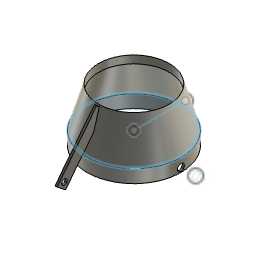
rudder (Autodesk Fusion 360 design; units mm, degrees)
Autodesk Fusion 360 part; units mm, degrees
note: some values were not read from the file. Chosen so that the rebuilt part matches the saved one: which bodies a step acts on.
sketch "Sketch1" plane through (0, 0, 0) normal (0, 0, 1) x (1, 0, 0) in component "Steering"
  circle A0 centre (-250, 0) radius 22
  line L0 (-250, 0) -> (-250, 24)
  circle A1 centre (-250, 0) radius 21
  dimension "d1" = 44
  dimension "d31" = 42
  constraint coincident A0.centre L0.start
  constraint vertical L0
  constraint concentric A0 A1
  measures "d1" diameter of A0
  measures "d31" diameter of A1
ref_plane "WorkPlane1" through (-225, 0, 0) normal (1, 0, 0) x (0, 1, 0) in component "Steering"
box "BoxPrimitive1" add length 30 width 1 height 5 placed x (0, 0, -1) y (-1, 0, 0) z (0, 1, 0) at (-254, 0, 23) makes body 1 in component "Steering"
move_body "Move1" bodies 1 to x (1, 0, 0) y (0, 0.906308, 0.422618) z (0, -0.422618, 0.906308) at (-0.9043, 30.3155, 9.0274) in component "Steering"
move_body "Move2" bodies 1 to x (1, 0, 0) y (0, 1, 0) z (0, 0, 1) at (2, 0, 0) in component "Steering"
move_body "Move3" bodies 1 to x (1, 0, 0) y (0, 1, 0) z (0, 0, 1) at (1.5, 0, 0) in component "Steering"
move_body "Move5" bodies 1 to x (1, 0, 0) y (0, 1, 0) z (0, 0, 1) at (1.9043, -35.5396, -3.7398) in component "Steering"
move_body "Move6" bodies 1 to x (1, 0, 0) y (0, 0.707107, -0.707107) z (0, 0.707107, 0.707107) at (0, -24.6397, 5.514) in component "Steering"
move_body "Move7" bodies 1 to x (1, 0, 0) y (0, 0.996195, -0.087156) z (0, 0.087156, 0.996195) at (0, -0.5088, 4.6655) in component "Steering"
move_body "Move8" bodies 1 to x (1, 0, 0) y (0, 1, 0) z (0, 0, 1) at (0, -9, 2) in component "Steering"
move_body "Move9" bodies 1 to x (1, 0, 0) y (0, 0.99863, -0.052336) z (0, 0.052336, 0.99863) at (0, -0.7634, -1.8095) in component "Steering"
hole "Hole1" at (-249.5, -32.4172, 16.2581) direction (-1, 0, 0) diameter 2.5 depth 1 tip angle 118 bodies 1 in component "Steering"
ref_plane "WorkPlane2" through (-21.1295, -2.354, 18.8882) normal (0, 0, 1) x (1, 0, 0) in component "Steering"
sketch "Sketch9" plane through (0, 0, 18.8882) normal (0, 0, 1) x (1, 0, 0) in component "Steering"
  circle A0 centre (-250, 0) radius 16.5
  dimension "d29" = 33
  measures "d29" diameter of A0
loft "Loft1" add profiles "Sketch9", "Sketch1" section 1 section 2 separate body makes body 2 in component "Steering"
shell "Shell1" thickness 1 removed faces 1 at (-244.1544, 9.3123, 0) on bodies 2 in component "Steering"
extrude "Extrude5" cut 1 faces at (-254.742, 5.5041, 18.8882) along direction (0, 0, -1) blind 10 on bodies 2 bodies 2 in component "Steering"
extrude "Extrude6" add sketch "Sketch1" against normal blind 6 bodies 2 in component "Steering"
move_body "Move14" bodies 1 to x (1, 0, 0) y (0, 0.984808, -0.173648) z (0, 0.173648, 0.984808) at (0, -7.8791, -30.8491) in component "Steering"
move_body "Move15" bodies 1 to x (1, 0, 0) y (0, 1, 0) z (0, 0, 1) at (0, 4, 5) in component "Steering"
split "Split2" by bodies 2 bodies 1 makes body 3 at (-249.5, -23.5105, 8.5052) makes body 4 at (-249.5, -15.6619, 16.4823) in component "Steering"
delete_body "RemoveBody2" bodies 4 in component "Steering"
ref_plane "WorkPlane3" through (-221.1295, -2.354, -6.1118) normal (1, 0, 0) x (0, 1, 0) in component "Steering"
sketch "Sketch17" plane through (-221.1295, 0, 0) normal (1, 0, 0) x (0, 1, 0) in component "Steering"
  circle A0 centre (0, -4) radius 1.6
  dimension "d37" = 3.2
  measures "d37" diameter of A0
extrude "Extrude7" cut sketch "Sketch17" against normal blind 57 bodies 2 in component "Steering"
component "Steering" placed x (1, 0, 0) y (0, 1, 0) z (0, 0, 1) at (21.1295, 2.354, 6.1118)
